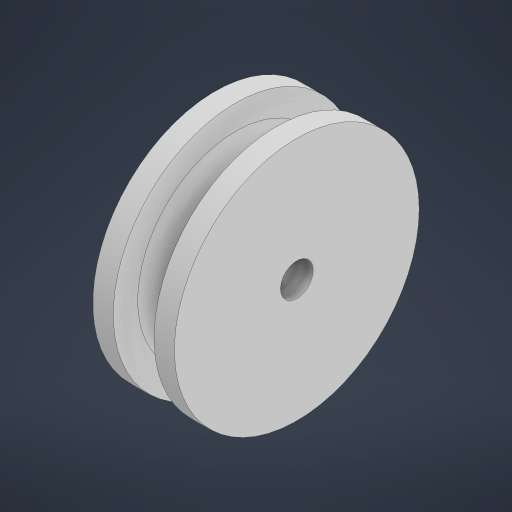
# Autodesk Inventor part: Align_Roller
Saved by Autodesk Inventor 2023 (Build 270158000, 158)
## iProperties
Created: 2023-11-08
Part Number: Align_Roller
Material: Generic
Document SubType Name: Modeling
Designer: Abhinav
Density: 1 g/cm^3
Appearance: Default
Author: Abhinav
Autodesk Inventor part; units mm, degrees
ref_plane "YZ Plane" through (0, 0, 0) normal (1, 0, 0) x (0, 1, 0)
ref_plane "XZ Plane" through (0, 0, 0) normal (0, 1, 0) x (-1, 0, 0)
ref_plane "XY Plane" through (0, 0, 0) normal (0, 0, 1) x (1, 0, 0)
sketch "Sketch1" plane through (0, 0, 0) normal (0, 1, 0) x (-1, 0, 0)
  line L0 (0, 0) -> (0, -10) construction
  line L1 (0, -10) -> (2.5, -10)
  line L2 (2.5, -10) -> (2.5, -15)
  line L3 (2.5, -15) -> (5, -15)
  line L4 (5, -15) -> (5, -2)
  line L5 (5, 0) -> (0, 0) construction
  line L6 (0, -10) -> (-2.5, -10)
  line L7 (-2.5, -10) -> (-2.5, -15)
  line L8 (-2.5, -15) -> (-5, -15)
  line L9 (-5, -15) -> (-5, -2)
  line L10 (-5, 0) -> (0, 0) construction
  line L11 (5, 0) -> (5, -2) construction
  line L12 (5, -2) -> (-5, -2)
  dimension "d1" = 10
  dimension "d2" = 2.5
  dimension "d3" = 5
  dimension "d4" = 2.5
  dimension "d7" = 2
  constraints: 26 end point, 6 perpendicular, 4 symmetric about line, 1 vertical
  measures "d1" distance of L0.start L0.end
  measures "d2" distance of L0.end L1.end
  measures "d3" distance of L1.end L2.end
  measures "d4" distance of L2.end L3.end
  measures "d7" distance of L4.end L5.start
revolve "Revolution1" add sketch "Sketch1" angle 360 about axis through (-5, 0, 0) along (1, 0, 0)
fillet "Fillet1" radius 2 2 edges at (-2.5, 0, 10) (2.5, 0, 10)
body "Solid1"
